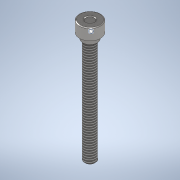
# Autodesk Inventor part: M2
Saved by Autodesk Inventor 2022.2 (Build 262287000, 287)
## iProperties
Created: 2022-08-20
Part Number: M2
Material: Steel, Galvanized
Document SubType Name: Modeling
Designer: ABL
Density: 7.85 g/cm^3
Appearance: Galvanized
Author: ABL
Autodesk Inventor part; units mm, degrees
ref_plane "YZ Plane" through (0, 0, 0) normal (1, 0, 0) x (0, 1, 0)
sketch "Sketch11" plane through (0, 0, 0) normal (0, 1, 0) x (-1, 0, 0)
  circle A0 centre (0, 0) radius 1.9
  dimension "d86" = 3.8
  constraints: 1 centre point, 1 coincident
  measures "d86" diameter of A0
sketch "Sketch12" plane through (0, 0, 0) normal (0, 1, 0) x (-1, 0, 0)
  circle A0 centre (0, 0) radius 1.3
  dimension "d87" = 2.6
  constraints: 1 centre point, 1 coincident
  measures "d87" diameter of A0
ref_plane "Work Plane4" through (0, 2, 0) normal (0, 1, 0) x (-1, 0, 0)
ref_plane "Work Plane5" through (0, 1.9, 0) normal (0, 1, 0) x (-1, 0, 0)
extrude "Head" add sketch "Sketch11" along normal blind 2
chamfer "Chamfer3" distance 0.1 angle 60 1 edges at (1.9, 2, 0) measured on face at (-1.8938, 1.3333, -0.1529)
sketch "Sketch6" plane through (0, 1.9, 0) normal (0, 1, 0) x (1, 0, 0)
  line L0 (0, 0) -> (-1.9, 0) construction
  line L1 (0, 0) -> (-2, 0) construction
  line L2 (-2, 0) -> (-2, 0.2)
  line L3 (-2, 0) -> (-2, -0.2)
  line L4 (-2, -0.2) -> (-1.8894, -0.2)
  line L5 (-2, 0.2) -> (-1.8894, 0.2)
  line L6 (-1.8894, -0.2) -> (-1.8894, 0.2)
  circle A0 centre (0, 0) radius 1.9 construction
  dimension "d34" = 1.9
  dimension "d35" = 2
  dimension "d36" = 0.2
  dimension "d37" = 0.2
  dimension "d40" = 0.1106
  dimension "d75" = 3.8
  constraints: 14 end point, 3 horizontal, 2 point on circle, 2 vertical, 1 centre point, 1 coincident, 1 perpendicular
  measures "d34" distance of L0.start L0.end
  measures "d35" distance of L0.start L1.end
  measures "d36" distance of L1.end L2.end
  measures "d37" distance of L1.end L3.end
  measures "d40" distance of L2.end L5.end
  measures "d75" diameter of A0
extrude "Grip Knurling" [suppressed]
fillet "Fillet3" [suppressed]
pattern_circular "Circular Pattern1" [suppressed]
pattern_circular "Circular Pattern2" [suppressed]
sketch "Label" plane through (0, 2, 0) normal (0, 1, 0) x (-1, 0, 0)
  circle A0 centre (0, 0) radius 0.866
  circle A1 centre (0, 0) radius 1.7268 projected
  dimension "shaftDiameter" = 2
  dimension "transitionDiameter" = 2.6
  dimension "d109" = 1.7321
  constraints: 1 centre point, 1 coincident, 1 other
  measures "d109" diameter of A0
feature "Bolt Designation" [suppressed]
sketch "Sketch2" plane through (0, 2, 0) normal (0, 1, 0) x (1, 0, 0)
  line L0 (0.75, -0.433) -> (0, -0.866)
  line L1 (0, -0.866) -> (-0.75, -0.433)
  line L2 (-0.75, -0.433) -> (-0.75, 0.433)
  line L3 (-0.75, 0.433) -> (0, 0.866)
  line L4 (0, 0.866) -> (0.75, 0.433)
  line L5 (0.75, 0.433) -> (0.75, -0.433)
  line L6 (-0.75, -0.433) -> (0.75, 0.433) construction
  point P0 (0, 0)
  point P1 (0, 0)
  dimension "d8" = 1.5
  dimension "d24" = 1.7321
  dimension "d85" = 0.866
  constraints: 14 end point, 1 coincident, 1 vertical, 13 other
  measures "d8" distance between parallel lines of L5 L2
  measures "d24" distance of L1.end L4.end
  measures "d85" distance of L0.start L0.end
extrude "HexagonSocket" [suppressed]
sketch "Sketch4" plane through (0, 2, 0) normal (0, 1, 0) x (1, 0, 0)
  circle A0 centre (0, 0) radius 0.866
  dimension "d25" = 1.7321
  constraints: 1 centre point, 1 coincident
  measures "d25" diameter of A0
extrude "Socket_topTaper" cut sketch "Sketch4" against normal blind 0.116 draft -45
ref_plane "Work Plane8" through (0, 0.8, 0) normal (0, 1, 0) x (1, 0, 0)
sketch "Sketch10" plane through (0, 0.8, 0) normal (0, 1, 0) x (1, 0, 0)
  circle A0 centre (0, 0) radius 0.433
  dimension "d70" = 0.866
  constraints: 1 centre point, 1 coincident
  measures "d70" diameter of A0
feature "Socket_bottomTaper" [suppressed]
extrude "Transition" add sketch "Sketch12" against normal blind 1
ref_plane "Work Plane9" through (0, -1, 0) normal (0, 1, 0) x (-1, 0, 0)
sketch "Sketch18" plane through (0, -1, 0) normal (0, -1, 0) x (1, 0, 0)
  circle A0 centre (0, 0) radius 1.3 projected
extrude "Extruded Angle" add sketch "Sketch18" along normal blind 0.2 draft -56.31
sketch "Sketch19" plane through (0, -1.2, 0) normal (0, -1, 0) x (1, 0, 0)
  circle A0 centre (0, 0) radius 1 projected
sketch "Sketch13" plane through (0, -1, 0) normal (0, -1, 0) x (1, 0, 0)
  circle A0 centre (0, 0) radius 1
  dimension "d92" = 2
  constraints: 1 centre point, 1 coincident
  measures "d92" diameter of A0
extrude "Shaft" add sketch "Sketch13" along normal blind 19
fillet "Fillet4" radius 0.2 1 edges at (1.3, 0, 0)
chamfer "Chamfer4" distance 0.2 angle 45 1 edges at (-1, -20, 0)
thread "Thread1" size "M2x0.4" class "6g" standard "ISO Metric profile" full length
sketch "Sketch7" plane through (0, 0, 0) normal (0, 0, 1) x (1, 0, 0)
  line L0 (-1, 0.2) -> (1, 0.2) construction
  line L1 (-1, -20.4) -> (-0.7393, -20.5505)
  line L2 (-0.7393, -20.6495) -> (-1, -20.8)
  line L3 (-1, -20.8) -> (-1, -20.4)
  arc A0 (-0.7393, -20.6495) -> (-0.7393, -20.5505) centre (-0.7679, -20.6) ccw
  line L4 (-1, -19.8) -> (1, -19.8) projected
  point P0 (0, 0)
  point P1 (-0.8845, -20.6)
  point P2 (-0.6536, -20.6)
  dimension "d53" = 0.4
  dimension "d56" = 0.0571
  dimension "d124" = 0.6
  dimension "d125" = 0
  constraints: 6 end point, 2 point on circle, 2 point on line, 2 tangent, 1 centre point, 1 vertical, 7 other
  measures "d53" distance of L2.end L1.start
  measures "d56" radius of A0
  measures "d124" distance from line of L4 L1.start
  measures "d125" horizontal distance of L4.start L1.start
feature "ModeledThreads" [suppressed]
extrude "Extrusion10" add sketch "Sketch19" against normal blind 1
equation "\"shaftDiameter\" = 2"
equation "\"transitionDiameter\" = 2.6"
equation "\"flangeCoupling_mountHoleDiameter\" = 3.9"
equation "\"headHeight\" = 2"
equation "\"headDiameter\" = 3.8"
equation "\"gap\" = 0.1"
equation "\"airgap\" = 0.4"
equation "\"wallgap\" = 2"
equation "\"printingLayerHeight\" = 0.2"
equation "\"driveMagnet_height\" = 5"
equation "\"halbachMagnet_height\" = 3"
equation "\"rotorBandBolt_diameter\" = 2"
equation "\"rotorBandBolt_headDiameter\" = 3.98"
equation "\"rotorBandBolt_headHeight\" = 2"
equation "\"rotorBandHexNut_sideToSide\" = 4"
equation "\"rotorBandHexNut_height\" = 1.2"
equation "\"rotorBandSquareNut_sideLength\" = 4"
equation "\"rotorBandSquareNut_height\" = 1.2"
equation "\"sensorMagnet_diameter\" = 5"
equation "\"sensorMagnet_height\" = 2.66667"
equation "\"sensorMagnet_ringRadius\" = 0.5 * driveMagnet_centerSpacingRadius + 2 * wallgap"
equation "\"rotorRadius\" = 2 * gap + driveMagnet_centerSpacingRadius + driveMagnet_length + wallgap"
equation "\"rotor_mountingLipHeight\" = 0.5 * statorThickness"
equation "\"flangeBearing_innerDiameter\" = shaftDiameter"
equation "\"flangeBearing_outerDiameter\" = 16"
equation "\"flangeBearing_flangeDiameter\" = 18"
equation "\"flangeBearing_height\" = 5"
equation "\"flangeBearing_flangeHeight\" = 1"
equation "\"magnetWire_outerDiameter\" = 0.8128"
equation "\"coilThickness\" = 12"
equation "\"statorThickness\" = coilThickness + 2 * wallgap"
equation "\"rotorBandThickness\" = wallgap + rotorBandBolt_headHeight + gap"
equation "\"flangeCoupling_innerDiameter\" = shaftDiameter"
equation "\"flangeCoupling_collarOuterDiameter\" = 16"
equation "\"flangeCoupling_flangeDiameter\" = 32"
equation "\"flangeCoupling_flangeHeight\" = 3.1"
equation "\"flangeCoupling_height\" = flangeCoupling_collarHeight + flangeCoupling_flangeHeight"
equation "\"flangeCoupling_mountHoleEdgeToEdge\" = 2.05"
equation "\"statorRadius\" = driveMagnet_length + driveMagnet_centerSpacingRadius + 2 * gap"
equation "\"statorMountBolt_diameter\" = 4"
equation "\"statorMountBolt_headDiameter\" = 7"
equation "\"statorMountBolt_headHeight\" = 4"
equation "\"statorMountBolt_shaftLength\" = coilThickness + flangeCoupling_flangeHeight + wallgap"
equation "\"statorMountHexNut_sideToSide\" = 8"
equation "\"statorMountHexNut_height\" = 4"
equation "\"coil_percentCoverage\" = 0.6"
equation "\"statorSpokeDegrees\" = 4deg"
equation "\"statorCoilBolt_diameter\" = 2"
equation "\"statorCoilBolt_headDiameter\" = 3.98"
equation "\"statorCoilBolt_headHeight\" = 2"
equation "\"statorCoilBolt_shaftLength\" = coilThickness"
equation "\"statorCoilHexNut_sideToSide\" = 4"
equation "\"statorCoilHexNut_height\" = 1.2"
equation "\"circuitBoard_height\" = 1.6"
equation "\"hallEffectSensor_height\" = 1.1"
equation "\"hallEffectSensor_length\" = 3"
equation "\"hallEffectSensor_width\" = 1.6"
equation "\"hallEffectSensor_pinLength\" = 0.6"
equation "\"circuitboardMountBolt_diameter\" = 2"
equation "\"circuitboardMountBolt_headDiameter\" = 3.98"
equation "\"circuitboardMountBolt_headHeight\" = 2"
equation "\"circuitboardMountBolt_shaftLength\" = coilThickness"
equation "\"circuitboardMountHexNut_sideToSide\" = 4"
equation "\"circuitboardMountHexNut_height\" = 1.2"
equation "\"statorShellBolt_diameter\" = 3"
equation "\"statorShellBolt_headDiameter\" = 5.68"
equation "\"statorShellBolt_headHeight\" = 3"
equation "\"statorShellBolt_shaftLength\" = statorThickness - statorShellBolt_countersinkDepth"
equation "\"statorShellHexNut_sideToSide\" = 5.3"
equation "\"statorShellHexNut_height\" = 2.3"
equation "\"threadPitch\" = 0.4"
equation "\"socketSize\" = 1.5"
equation "\"chamferSize\" = 0.2"
equation "\"keyEngagementDepth\" = 1"
equation "\"transitionLength\" = 1"
equation "\"textSize\" = 0.95"
equation "\"driveMagnet_centerSpacingRadius\" = 38.96113"
equation "\"driveMagnet_length\" = 60"
equation "\"flangeCoupling_collarHeight\" = 10"
equation "\"statorShellBolt_countersinkDepth\" = 3.4"
body "Solid17"
